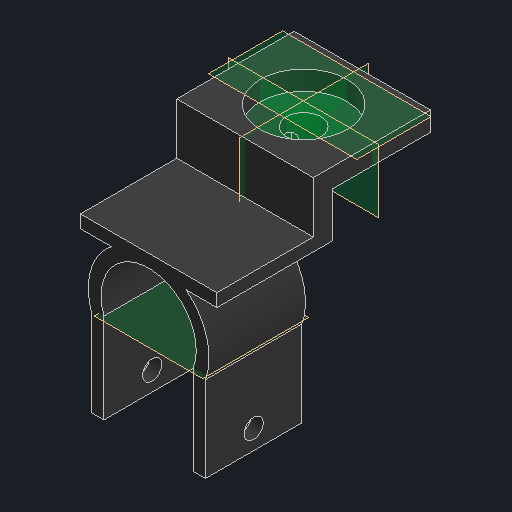
# Autodesk Inventor part: camera_base
Saved by Autodesk Inventor 2026.1 (Build 301233020, 233B)
## iProperties
Created: 2025-12-04
Part Number: camera_base
Material: 고무, 검은색
Document SubType Name: Modeling
Designer: jaewook
Density: 0.93 g/cm^3
Appearance: 고무 - 검은색
Author: jaewook
Autodesk Inventor part; units mm, degrees
ref_plane "YZ Plane" through (0, 0, 0) normal (1, 0, 0) x (0, 1, 0)
ref_plane "XZ Plane" through (0, 0, 0) normal (0, 1, 0) x (-1, 0, 0)
ref_plane "XY Plane" through (0, 0, 0) normal (0, 0, 1) x (1, 0, 0)
ref_plane "작업 평면1" through (-110.7617, -266.6078, -340.9184) normal (0, -1, 0) x (1, 0, 0)
sketch "스케치1" plane through (-110.7617, -266.6078, -340.9184) normal (0, -1, 0) x (1, 0, 0)
  circle A0 centre (21.5, 10.75) radius 6.45 projected
  circle A1 centre (21.5, 10.75) radius 2.3 projected
  line L0 (10.8797, 19.8723) -> (32.1203, 19.8723)
  line L1 (32.1203, 19.8723) -> (32.1203, 1.6277)
  line L2 (32.1203, 1.6277) -> (10.8797, 1.6277)
  line L3 (10.8797, 1.6277) -> (10.8797, 19.8723)
  line L4 (10.8797, 19.8723) -> (32.1203, 1.6277) construction
  line L5 (32.1203, 19.8723) -> (10.8797, 1.6277) construction
  circle A2 centre (21.5, 10.75) radius 6.75
  point P0 (110.7617, 340.9184)
  dimension "d37" = 0.3
  constraints: 12 end point, 2 midpoint, 2 parallel, 1 centre point, 1 horizontal, 1 perpendicular
  measures "d37" radial gap between concentric circles of A0 A2
extrude "돌출1" add sketch "스케치1" along normal blind 3 contours L0 L1 L2 L3
ref_plane "작업 평면2" through (-89.2617, -269.6078, -330.1684) normal (0, -1, 0) x (1, 0, 0)
sketch "스케치3" plane through (-110.7617, -269.6078, -340.9184) normal (0, -1, 0) x (1, 0, 0)
  circle A0 centre (21.5, 10.75) radius 2.3 projected
  circle A1 centre (21.5, 10.75) radius 2.3 projected
  circle A2 centre (21.5, 10.75) radius 7.25
  circle A3 centre (21.5, 10.75) radius 2.7
  circle A4 centre (21.5, 10.75) radius 6.75 projected
  circle A5 centre (21.5, 10.75) radius 6.75 projected
  point P0 (110.7617, 340.9184)
  dimension "d5" = 0.4
  dimension "d38" = 0.5
  constraints: 2 centre point
  measures "d5" radial gap between concentric circles of A0 A3
  measures "d38" radial gap between concentric circles of A4 A2
extrude "돌출2" add sketch "스케치3" along normal blind 1 contours A2 | A4
sketch "스케치4" plane through (-89.2617, -270.6078, -330.1684) normal (0, -1, 0) x (1, 0, 0)
  circle A0 centre (0, 0) radius 2.7 projected
  circle A1 centre (0, 0) radius 3.7
  circle A2 centre (0, 0) radius 3
  point P0 (89.2617, 330.1684)
  dimension "d6" = 1
  dimension "d41" = 0.3
  constraints: 2 centre point
  measures "d6" radial gap between concentric circles of A0 A1
  measures "d41" radial gap between concentric circles of A0 A2
extrude "돌출3" add sketch "스케치4" along normal blind 4.1 contours A1 | A2
sketch "스케치6" plane through (-89.2617, -274.7078, -330.1684) normal (0, -1, 0) x (1, 0, 0)
  circle A0 centre (0, 0) radius 3.7 projected
  point P0 (89.2617, 330.1684)
extrude "돌출4" add sketch "스케치6" along normal blind 0.9
ref_plane "작업 평면7" through (-78.6413, -266.6078, -330.1684) normal (0, 0, -1) x (-1, 0, 0)
sketch "스케치7" plane through (-78.6413, -266.6078, -330.1684) normal (0, 0, -1) x (-1, 0, 0)
  line L0 (6.9203, -4) -> (6.9203, -9) projected
  line L1 (14.3203, -4) -> (14.3203, -9) projected
  line L2 (6.9203, -9) -> (14.3203, -9) projected
  line L3 (6.9203, -8.2) -> (14.3203, -8.2)
  line L4 (14.3203, -8.2) -> (14.3203, -6.7)
  line L5 (14.3203, -6.7) -> (6.9203, -6.7)
  line L6 (6.9203, -6.7) -> (6.9203, -8.2)
  point P0 (-78.6413, 266.6078)
  dimension "d15" = 0.8
  dimension "d16" = 3
  constraints: 8 end point, 2 parallel, 2 point on line, 1 horizontal, 1 perpendicular
  measures "d15" distance between parallel lines of L3 L2
  measures "d16" diameter of L3 L5
revolve "회전2" cut sketch "스케치7" angle 360 about axis through (-92.9617, -273.3078, -330.1684) along (1, 0, 0) contours L5 L1 L3 L0
sketch "스케치8" plane through (-110.7617, -269.6078, -340.9184) normal (0, -1, 0) x (1, 0, 0)
  line L0 (32.1203, 1.6277) -> (32.1203, 19.8723) projected
  line L1 (32.1203, 19.8723) -> (10.8797, 19.8723) projected
  line L2 (10.8797, 19.8723) -> (10.8797, 1.6277) projected
  line L3 (10.8797, 16.8723) -> (32.1203, 16.8723)
  line L4 (32.1203, 16.8723) -> (32.1203, 19.8723)
  line L5 (32.1203, 19.8723) -> (10.8797, 19.8723)
  line L6 (10.8797, 19.8723) -> (10.8797, 16.8723)
  point P0 (110.7617, 340.9184)
  point P1 (32.1203, 16.8723)
  dimension "d18" = 3
  constraints: 8 end point, 2 parallel, 1 horizontal, 1 perpendicular, 1 point on line
  measures "d18" distance between parallel lines of L1 L3
extrude "돌출5" add sketch "스케치8" along normal blind 7
ref_plane "작업 평면8" through (-89.2617, -266.6078, -339.2906) normal (-1, 0, 0) x (0, 0, 1)
sketch "스케치9" plane through (-89.2617, -266.6078, -339.2906) normal (-1, 0, 0) x (0, 0, 1)
  line L0 (18.2445, 0) -> (18.2445, -10) projected
  line L1 (18.2445, -10) -> (33.2445, -10)
  line L2 (33.2445, -10) -> (33.2445, -17.4)
  line L3 (33.2445, -17.4) -> (18.2445, -17.4)
  line L4 (18.2445, -17.4) -> (18.2445, -10)
  line L5 (18.2445, -10) -> (18.2445, -8)
  line L6 (33.2445, -8) -> (18.2445, -8)
  line L7 (33.2445, -8) -> (33.2445, -10)
  point P0 (339.2906, 266.6078)
  dimension "d21" = 14.8
  dimension "d22" = 15
  dimension "d23" = 2
  constraints: 14 end point, 3 perpendicular, 2 parallel, 1 horizontal, 1 point on line
  measures "d21" diameter of L1 L3
  measures "d22" distance of L0.end L1.end
  measures "d23" distance of L6.start L1.end
revolve "회전3" add sketch "스케치9" angle 220 mid plane about axis through (-89.2617, -284.0078, -306.0461) along (0, 0, -1) contours L6 L7 L1 L0
sketch "스케치11" plane through (-99.882, -266.6078, -321.0461) normal (0, 0, 1) x (1, 0, 0)
  arc A0 (16.4169, -10) -> (4.8238, -10) centre (10.6203, -17.4) ccw projected
  line L0 (21.2407, 0) -> (21.2407, -10) projected
  line L1 (0, 0) -> (0, -10) projected
  line L2 (4.8238, -10) -> (0, -10) projected
  line L3 (0, -8) -> (21.2407, -8)
  point P0 (99.882, 266.6078)
  point P1 (10.6203, -8)
  constraints: 2 end point, 2 point on line, 1 perpendicular
extrude "돌출7" add sketch "스케치11" along normal up to surface (15 mm away)
mirror "미러1" about plane through (-89.2617, -266.6078, -339.2906) normal (-1, 0, 0) of "돌출7"
ref_plane "작업 평면9" through (-96.2154, -286.5387, -306.0461) normal (0, -1, 0) x (0, 0, -1)
sketch "스케치12" plane through (-96.2154, -286.5387, -306.0461) normal (0, -1, 0) x (0, 0, -1)
  line L0 (0, -1.8794) -> (15, -1.8794) projected
  line L1 (15, -1.8794) -> (15, 0) projected
  line L2 (15, 0) -> (0, 0) projected
  line L3 (0, 0) -> (0, -1.8794) projected
  line L4 (15, 15.7868) -> (0, 15.7868) projected
  line L5 (0, 15.7868) -> (0, 13.9075) projected
  line L6 (0, 13.9075) -> (15, 13.9075) projected
  line L7 (15, 13.9075) -> (15, 15.7868) projected
  point P0 (-306.0461, 96.2154)
extrude "돌출8" add sketch "스케치12" along normal blind 14
sketch "스케치13" plane through (-98.0948, -287.2228, -321.0461) normal (-1, 0, 0) x (0, 0, 1)
  circle A0 centre (7.5, -10.316) radius 1.5
  line L0 (15, -13.316) -> (0, -13.316) projected
  line L1 (15, 0) -> (15, -13.316) projected
  point P0 (321.0461, 287.2228)
  dimension "d34" = 3
  dimension "d39" = 3
  dimension "d40" = 7.5
  constraints: 1 centre point
  measures "d34" diameter of A0
  measures "d39" distance from line of A0.centre L0
  measures "d40" distance from line of L1 A0.centre
extrude "돌출9" cut sketch "스케치13" against normal through all
